Autodesk Fusion 360 part; units mm, degrees
(part 2 of 4)
sketch "Sketch2" plane through (-153, -3, 890) normal (0, -1, 0) x (1, 0, 0)
  circle A0 centre (0, 0) radius 2.75
  circle A1 centre (0, 0) radius 2.75
  circle A2 centre (81, 0) radius 2.75
  circle A3 centre (81, 0) radius 2.75
  circle A4 centre (162, 0) radius 2.75
  circle A5 centre (243, 0) radius 2.75
  circle A6 centre (243, 0) radius 2.75
  circle A7 centre (162, 0) radius 2.75
  circle A8 centre (405, 0) radius 2.75
  circle A9 centre (405, 0) radius 2.75
  circle A10 centre (324, 0) radius 2.75
  circle A11 centre (324, 0) radius 2.75
  circle A12 centre (486, 0) radius 2.75
  circle A13 centre (486, 0) radius 2.75
  circle A14 centre (405, -81) radius 2.75
  circle A15 centre (81, -81) radius 2.75
  circle A16 centre (486, -81) radius 2.75
  circle A17 centre (405, -81) radius 2.75
  circle A18 centre (0, -81) radius 2.75
  circle A19 centre (0, -81) radius 2.75
  circle A20 centre (81, -81) radius 2.75
  circle A21 centre (324, -81) radius 2.75
  circle A22 centre (243, -81) radius 2.75
  circle A23 centre (486, -81) radius 2.75
  circle A24 centre (243, -81) radius 2.75
  circle A25 centre (324, -81) radius 2.75
  circle A26 centre (162, -81) radius 2.75
  circle A27 centre (162, -81) radius 2.75
  circle A28 centre (162, -162) radius 2.75
  circle A29 centre (162, -243) radius 2.75
  circle A30 centre (81, -243) radius 2.75
  circle A31 centre (162, -162) radius 2.75
  circle A32 centre (162, -243) radius 2.75
  circle A33 centre (324, -243) radius 2.75
  circle A34 centre (81, -162) radius 2.75
  circle A35 centre (324, -162) radius 2.75
  circle A36 centre (243, -243) radius 2.75
  circle A37 centre (405, -162) radius 2.75
  circle A38 centre (486, -243) radius 2.75
  circle A39 centre (81, -162) radius 2.75
  circle A40 centre (81, -243) radius 2.75
  circle A41 centre (405, -243) radius 2.75
  circle A42 centre (0, -162) radius 2.75
  circle A43 centre (243, -162) radius 2.75
  circle A44 centre (405, -162) radius 2.75
  circle A45 centre (486, -162) radius 2.75
  circle A46 centre (0, -243) radius 2.75
  circle A47 centre (486, -162) radius 2.75
  circle A48 centre (243, -162) radius 2.75
  circle A49 centre (0, -162) radius 2.75
  circle A50 centre (0, -243) radius 2.75
  circle A51 centre (243, -243) radius 2.75
  circle A52 centre (324, -162) radius 2.75
  circle A53 centre (405, -243) radius 2.75
  circle A54 centre (324, -243) radius 2.75
  circle A55 centre (486, -243) radius 2.75
  circle A56 centre (486, -324) radius 2.75
  circle A57 centre (243, -324) radius 2.75
  circle A58 centre (405, -324) radius 2.75
  circle A59 centre (81, -324) radius 2.75
  circle A60 centre (324, -324) radius 2.75
  circle A61 centre (0, -324) radius 2.75
  circle A62 centre (405, -324) radius 2.75
  circle A63 centre (486, -324) radius 2.75
  circle A64 centre (81, -324) radius 2.75
  circle A65 centre (162, -324) radius 2.75
  circle A66 centre (243, -324) radius 2.75
  circle A67 centre (162, -324) radius 2.75
  circle A68 centre (324, -324) radius 2.75
  circle A69 centre (0, -324) radius 2.75
  point P0 (81, 0)
  point P1 (81, 0)
  point P2 (162, 0)
  point P3 (243, 0)
  point P4 (324, 0)
  point P5 (405, 0)
  point P6 (486, 0)
  point P7 (162, 0)
  point P8 (243, 0)
  point P9 (243, 0)
  point P10 (324, 0)
  point P11 (405, 0)
  point P12 (405, 0)
  point P13 (324, 0)
  point P14 (405, 0)
  point P15 (486, 0)
  point P16 (486, 0)
  point P17 (486, 0)
  point P18 (486, 0)
  point P19 (0, -81)
  point P20 (0, -162)
  point P21 (0, -243)
  point P22 (0, -324)
  point P23 (162, -81)
  point P24 (243, -81)
  point P25 (0, -81)
  point P26 (243, -81)
  point P27 (324, -81)
  point P28 (405, -81)
  point P29 (81, -81)
  point P30 (486, -81)
  point P31 (324, -81)
  point P32 (405, -81)
  point P33 (405, -81)
  point P34 (324, -81)
  point P35 (162, -81)
  point P36 (243, -81)
  point P37 (486, -81)
  point P38 (486, -81)
  point P39 (486, -81)
  point P40 (486, -81)
  point P41 (405, -81)
  point P42 (81, -81)
  point P43 (405, -243)
  point P44 (324, -243)
  point P45 (243, -243)
  point P46 (405, -243)
  point P47 (486, -243)
  point P48 (486, -243)
  point P49 (162, -243)
  point P50 (324, -243)
  point P51 (81, -243)
  point P52 (81, -243)
  point P53 (162, -243)
  point P54 (405, -243)
  point P55 (405, -243)
  point P56 (243, -243)
  point P57 (0, -243)
  point P58 (324, -243)
  point P59 (486, -243)
  point P60 (486, -243)
  point P61 (486, -243)
  point P62 (243, -243)
  point P63 (162, -162)
  point P64 (243, -162)
  point P65 (0, -162)
  point P66 (243, -162)
  point P67 (324, -162)
  point P68 (0, -243)
  point P69 (405, -162)
  point P70 (81, -162)
  point P71 (486, -162)
  point P72 (324, -162)
  point P73 (405, -162)
  point P74 (405, -162)
  point P75 (324, -162)
  point P76 (162, -162)
  point P77 (243, -162)
  point P78 (486, -162)
  point P79 (486, -162)
  point P80 (486, -162)
  point P81 (486, -162)
  point P82 (405, -162)
  point P83 (81, -162)
  point P84 (0, -324)
  point P85 (0, -324)
  point P86 (486, -324)
  point P87 (0, -324)
  point P88 (162, -324)
  point P89 (81, -324)
  point P90 (486, -324)
  point P91 (486, -324)
  point P92 (243, -324)
  point P93 (405, -324)
  point P94 (486, -324)
  point P95 (162, -324)
  point P96 (81, -324)
  point P97 (405, -324)
  point P98 (243, -324)
  point P99 (324, -324)
  point P100 (486, -324)
  point P101 (324, -324)
  point P102 (405, -324)
  point P103 (324, -324)
  point P104 (405, -324)
  point P105 (243, -324)
  dimension "d286" = 5.5
  dimension "d287" = 5.5
  dimension "d288" = 5.5
  dimension "d289" = 5.5
  dimension "d290" = 5.5
  dimension "d291" = 5.5
  dimension "d292" = 5.5
  dimension "d293" = 5.5
  dimension "d294" = 5.5
  dimension "d295" = 5.5
  dimension "d296" = 5.5
  dimension "d297" = 5.5
  dimension "d298" = 5.5
  dimension "d299" = 5.5
  dimension "d300" = 5.5
  dimension "d301" = 5.5
  dimension "d302" = 5.5
  dimension "d303" = 5.5
  dimension "d304" = 5.5
  dimension "d305" = 5.5
  dimension "d306" = 5.5
  dimension "d307" = 5.5
  dimension "d308" = 5.5
  dimension "d309" = 5.5
  dimension "d310" = 5.5
  dimension "d311" = 5.5
  dimension "d312" = 5.5
  dimension "d313" = 5.5
  dimension "d314" = 5.5
  dimension "d315" = 5.5
  dimension "d316" = 5.5
  dimension "d317" = 5.5
  dimension "d318" = 5.5
  dimension "d319" = 5.5
  dimension "d320" = 5.5
  dimension "d321" = 5.5
  dimension "d322" = 5.5
  dimension "d323" = 5.5
  dimension "d324" = 5.5
  dimension "d325" = 5.5
  dimension "d326" = 5.5
  dimension "d327" = 5.5
  dimension "d328" = 5.5
  dimension "d329" = 5.5
  dimension "d330" = 5.5
  dimension "d331" = 5.5
  dimension "d332" = 5.5
  dimension "d333" = 5.5
  dimension "d334" = 5.5
  dimension "d335" = 5.5
  dimension "d336" = 5.5
  dimension "d337" = 5.5
  dimension "d338" = 5.5
  dimension "d339" = 5.5
  dimension "d340" = 5.5
  dimension "d341" = 5.5
  dimension "d342" = 5.5
  dimension "d343" = 5.5
  dimension "d344" = 5.5
  dimension "d345" = 5.5
  dimension "d346" = 5.5
  dimension "d347" = 5.5
  dimension "d348" = 5.5
  dimension "d349" = 5.5
  dimension "d350" = 5.5
  dimension "d351" = 5.5
  dimension "d352" = 5.5
  dimension "d353" = 5.5
  dimension "d354" = 5.5
  dimension "d355" = 5.5
  constraint coincident A0.centre A1.centre
  constraint coincident P1 P0
  constraint coincident P7 P2
  constraint coincident P9 P8
  constraint coincident P13 P10
  constraint coincident P14 P12
  constraint coincident P18 P17
  constraint coincident P25 P19
  constraint coincident P42 P29
  constraint coincident P35 P23
  constraint coincident P36 P26
  constraint coincident P34 P31
  constraint coincident P41 P33
  constraint coincident P40 P39
  constraint coincident P65 P20
  constraint coincident P83 P70
  constraint coincident P76 P63
  constraint coincident P77 P66
  constraint coincident P75 P72
  constraint coincident P82 P74
  constraint coincident P81 P80
  constraint coincident P68 P57
  constraint coincident P52 P51
  constraint coincident P53 P49
  constraint coincident P62 P56
  constraint coincident P58 P50
  constraint coincident P55 P54
  constraint coincident P61 P60
  constraint coincident P87 P85
  constraint coincident P96 P89
  constraint coincident P95 P88
  constraint coincident P105 P98
  constraint coincident P103 P101
  constraint coincident P104 P102
  constraint coincident P100 P94
  measures "d286" diameter of A0
  measures "d287" diameter of A1
  measures "d288" diameter of A2
  measures "d289" diameter of A3
  measures "d290" diameter of A7
  measures "d291" diameter of A4
  measures "d292" diameter of A6
  measures "d293" diameter of A5
  measures "d294" diameter of A10
  measures "d295" diameter of A11
  measures "d296" diameter of A8
  measures "d297" diameter of A9
  measures "d298" diameter of A12
  measures "d299" diameter of A13
  measures "d300" diameter of A19
  measures "d301" diameter of A18
  measures "d302" diameter of A15
  measures "d303" diameter of A20
  measures "d304" diameter of A27
  measures "d305" diameter of A26
  measures "d306" diameter of A24
  measures "d307" diameter of A22
  measures "d308" diameter of A25
  measures "d309" diameter of A21
  measures "d310" diameter of A14
  measures "d311" diameter of A17
  measures "d312" diameter of A16
  measures "d313" diameter of A23
  measures "d314" diameter of A42
  measures "d315" diameter of A49
  measures "d316" diameter of A39
  measures "d317" diameter of A34
  measures "d318" diameter of A28
  measures "d319" diameter of A31
  measures "d320" diameter of A43
  measures "d321" diameter of A48
  measures "d322" diameter of A52
  measures "d323" diameter of A35
  measures "d324" diameter of A37
  measures "d325" diameter of A44
  measures "d326" diameter of A47
  measures "d327" diameter of A45
  measures "d328" diameter of A50
  measures "d329" diameter of A46
  measures "d330" diameter of A40
  measures "d331" diameter of A30
  measures "d332" diameter of A32
  measures "d333" diameter of A29
  measures "d334" diameter of A51
  measures "d335" diameter of A36
  measures "d336" diameter of A33
  measures "d337" diameter of A54
  measures "d338" diameter of A41
  measures "d339" diameter of A53
  measures "d340" diameter of A55
  measures "d341" diameter of A38
  measures "d342" diameter of A69
  measures "d343" diameter of A61
  measures "d344" diameter of A59
  measures "d345" diameter of A64
  measures "d346" diameter of A67
  measures "d347" diameter of A65
  measures "d348" diameter of A57
  measures "d349" diameter of A66
  measures "d350" diameter of A68
  measures "d351" diameter of A60
  measures "d352" diameter of A62
  measures "d353" diameter of A58
  measures "d354" diameter of A56
  measures "d355" diameter of A63
extrude "Extrude2" [suppressed]

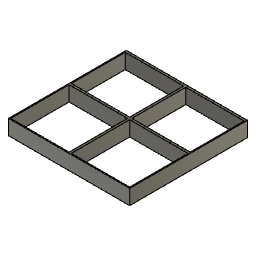
design "Grilla A."
Autodesk Fusion 360 part; units mm, degrees
ref_plane "WorkPlane1" through (0, 0, 0) normal (0, 0, 1) x (1, 0, 0)
sketch "Sketch1" plane through (0, 0, 0) normal (0, 0, 1) x (1, 0, 0)
  line L0 (39, 36.035) -> (-39, 36.035)
  line L1 (-39, 36.035) -> (-39, -36.035)
  line L2 (-39, -36.035) -> (39, -36.035)
  line L3 (39, -36.035) -> (39, 36.035)
  line L4 (39, 36.035) -> (-39, -36.035) construction
  line L5 (-39, 36.035) -> (39, -36.035) construction
  line L6 (-39, -36.035) -> (39, -36.035)
  line L7 (39, -39.035) -> (-39, -39.035)
  line L8 (-39, -39.035) -> (39, -39.035)
  line L9 (39, -39.035) -> (39, -117.035)
  line L10 (39, -117.035) -> (-39, -117.035)
  line L11 (-39, -117.035) -> (-39, -39.035)
  line L12 (120, 36.035) -> (42, -36.035) construction
  line L13 (120, -39.035) -> (120, -117.035)
  line L14 (42, -36.035) -> (120, -36.035)
  line L15 (42, -39.035) -> (120, -39.035)
  line L16 (120, -39.035) -> (42, -39.035)
  line L17 (120, -117.035) -> (42, -117.035)
  line L18 (42, -36.035) -> (120, -36.035)
  line L19 (42, -117.035) -> (42, -39.035)
  line L20 (120, 36.035) -> (42, 36.035)
  line L21 (42, 36.035) -> (42, -36.035)
  line L22 (120, -36.035) -> (120, 36.035)
  line L23 (42, 36.035) -> (120, -36.035) construction
  line L24 (120, 39.035) -> (-39, 39.035)
  line L25 (-39, 39.035) -> (-40.5, 39.035)
  line L26 (-40.5, 39.035) -> (-40.5, -117.035)
  line L27 (120, 39.035) -> (121.5, 39.035)
  line L28 (121.5, 39.035) -> (121.5, -117.035)
  line L29 (121.5, -117.035) -> (121.5, -118.535)
  line L30 (121.5, -118.535) -> (-40.5, -118.535)
  line L31 (-40.5, -118.535) -> (-40.5, -117.035)
  line L32 (-39, 36.035) -> (39, 36.035)
  line L33 (42, 36.035) -> (120, 36.035)
  line L34 (-39, -117.035) -> (-39, -39.035)
  line L35 (-39, -36.035) -> (-39, 36.035)
  line L36 (39, -117.035) -> (39, -39.035)
  line L37 (39, -36.035) -> (39, 36.035)
  line L38 (42, 36.035) -> (42, -36.035)
  line L39 (42, -39.035) -> (42, -117.035)
  line L40 (120, -117.035) -> (120, -39.035)
  line L41 (120, -36.035) -> (120, 36.035)
  line L42 (-39, -117.035) -> (39, -117.035)
  line L43 (42, -117.035) -> (120, -117.035)
  point P0 (81, 0)
  point P1 (81, 0)
  dimension "d55" = 78
  dimension "d56" = 72.07
  dimension "d57" = 3
  dimension "d58" = 78
  dimension "d59" = 78
  dimension "d60" = 78
  dimension "d61" = 72.07
  dimension "d62" = 3
  dimension "d63" = 78
  dimension "d64" = 78
  dimension "d65" = 3
  dimension "d66" = 3
  dimension "d67" = 1.5
  dimension "d68" = 1.5
  dimension "d69" = 1.5
  constraint horizontal L0
  constraint perpendicular L0 L1
  constraint parallel L0 L2
  constraint parallel L1 L3
  constraint coincident L4 origin
  constraint coincident L5 origin
  constraint horizontal L6
  constraint horizontal L7
  constraint horizontal L8
  constraint vertical L9
  constraint horizontal L10
  constraint vertical L11
  constraint horizontal L20
  constraint perpendicular L20 L21
  constraint parallel L18 L20
  constraint parallel L21 L22
  constraint coincident P1 L12
  constraint coincident P1 L23
  constraint coincident P1 P0
  constraint horizontal L14
  constraint horizontal L16
  constraint horizontal L15
  constraint vertical L13
  constraint horizontal L17
  constraint vertical L19
  constraint vertical L38
  constraint vertical L36
  constraint horizontal L32
  constraint horizontal L24
  constraint horizontal L25
  constraint vertical L26
  constraint vertical L34
  constraint horizontal L27
  constraint vertical L28
  constraint vertical L40
  constraint horizontal L42
  constraint vertical L29
  constraint horizontal L30
  constraint vertical L31
  constraint collinear L32 L33
  constraint collinear L34 L35
  constraint collinear L36 L37
  constraint collinear L38 L39
  constraint collinear L40 L41
  constraint collinear L42 L43
  measures "d55" distance of L1.end L2.end
  measures "d56" distance of L0.end L1.end
  measures "d57" distance of L1.end L7.end
  measures "d58" distance of L7.end L7.start
  measures "d59" distance of L7.end L10.end
  measures "d60" distance of L12.end L14.end
  measures "d61" distance of L20.end L12.end
  measures "d62" distance of L12.end L15.start
  measures "d63" distance of L15.start L13.start
  measures "d64" distance of L15.start L17.end
  measures "d65" distance of L0.start L20.end
  measures "d66" distance of L0.end L24.end
  measures "d67" distance of L24.end L25.end
  measures "d68" distance of L24.start L27.end
  measures "d69" distance of L26.end L30.end
extrude "Extrude2" add sketch "Sketch1" along normal blind 20

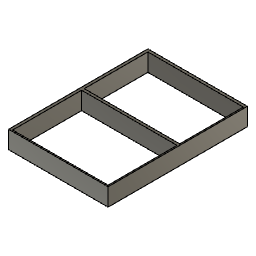
design "C Grilla"
Autodesk Fusion 360 part; units mm, degrees
sketch "Sketch1" plane through (0, 0, 0) normal (0, 0, 1) x (1, 0, 0)
  line L0 (54, 36) -> (-54, 36)
  line L1 (-54, 36) -> (-54, -36)
  line L2 (-54, -36) -> (54, -36)
  line L3 (54, -36) -> (54, 36)
  line L4 (54, 36) -> (-54, -36) construction
  line L5 (-54, 36) -> (54, -36) construction
  line L6 (-54, -39) -> (54, -39)
  line L7 (55.5, 39) -> (-57, 39)
  line L8 (-57, 39) -> (-57, -39)
  line L9 (-54, -39) -> (54, -39)
  line L10 (54, -39) -> (54, -117)
  line L11 (54, -117) -> (-54, -117)
  line L12 (-54, -117) -> (-54, -39)
  line L13 (-57, -39) -> (-57, -118.5)
  line L14 (55.5, -36) -> (55.5, 36)
  line L15 (55.5, -39) -> (55.5, -118.5)
  line L16 (55.5, -118.5) -> (-54, -118.5)
  line L17 (55.5, -36) -> (55.5, -39)
  line L18 (55.5, 36) -> (55.5, 39)
  line L19 (-54, -118.5) -> (-57, -118.5)
  dimension "d13" = 108
  dimension "d14" = 72
  dimension "d16" = 108
  dimension "d17" = 78
  dimension "d18" = 1.5
  dimension "d19" = -1.5
  constraint horizontal L0
  constraint perpendicular L0 L1
  constraint parallel L0 L2
  constraint parallel L1 L3
  constraint coincident L4 origin
  constraint coincident L5 origin
  constraint horizontal L9
  constraint vertical L10
  constraint horizontal L11
  constraint vertical L12
  constraint coincident L6.start L9.start
  constraint perpendicular L11 L13
  constraint parallel L2 L6
  constraint parallel L0 L7
  constraint parallel L1 L8
  constraint parallel L15 L17
  constraint perpendicular L7 L18
  constraint perpendicular L13 L19
  measures "d13" distance of L1.end L2.end
  measures "d14" distance of L0.end L1.end
  measures "d16" distance of L6.start L6.end
  measures "d17" distance of L6.start L11.end
extrude "Extrude2" add sketch "Sketch1" along normal blind 20

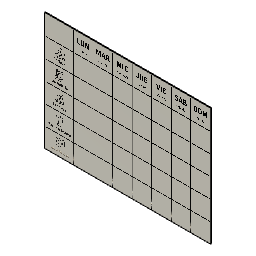
design "pantalla render"
Autodesk Fusion 360 part; units mm, degrees
sketch "Sketch1" plane through (0, 0, 0) normal (0, 1, 0) x (1, 0, 0)
  line L0 (340.5, 241.5) -> (-340.5, 241.5)
  line L1 (-340.5, 241.5) -> (-340.5, -241.5)
  line L2 (-340.5, -241.5) -> (340.5, -241.5)
  line L3 (340.5, -241.5) -> (340.5, 241.5)
  line L4 (340.5, 241.5) -> (-340.5, -241.5) construction
  line L5 (-340.5, 241.5) -> (340.5, -241.5) construction
  dimension "d1" = 681
  dimension "d2" = 483
  constraint horizontal L0
  constraint perpendicular L0 L1
  constraint parallel L0 L2
  constraint parallel L1 L3
  constraint coincident L4 origin
  constraint coincident L5 origin
  measures "d1" distance of L1.end L2.end
  measures "d2" distance of L0.end L1.end
extrude "Extrude1" add sketch "Sketch1" against normal blind 3

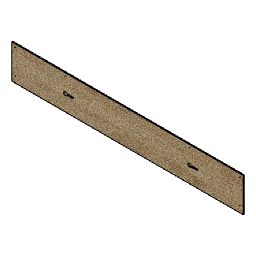
design "Pieza trasera fondo"
Autodesk Fusion 360 part; units mm, degrees
sketch "Sketch1" plane through (0, 0, 0) normal (0, 1, 0) x (1, 0, 0)
  arc A0 (187.942, -190.4984) -> (187.4765, -190.7709) centre (187.922, -190.998) ccw
  line L0 (340.5, -50) -> (337.5, -50)
  line L1 (-161.02, -186.5) -> (-178.0217, -186.5)
  circle A1 centre (330.5, -232.5) radius 1
  line L2 (188.022, -190.5) -> (205.0238, -190.5)
  line L3 (-337.5, -238.5) -> (-340.5, -238.5)
  circle A2 centre (183.022, -233.5) radius 1
  arc A3 (187.942, -190.4984) -> (188.022, -190.5) centre (188.022, -188.5) ccw
  line L4 (50, -238.5) -> (50, -241.5)
  line L5 (-337.5, -238.5) -> (-337.5, -241.5)
  arc A4 (187.4765, -186.2291) -> (187.942, -186.5016) centre (187.922, -186.002) ccw
  circle A5 centre (-183.0217, -233.5) radius 1
  circle A6 centre (328.5, 226.5) radius 1
  circle A7 centre (330.5, -159.5) radius 1
  circle A8 centre (-330.5, -232.5) radius 1
  line L6 (50, 238.5) -> (337.5, 238.5)
  line L7 (-337.5, 50) -> (-337.5, 238.5)
  circle A9 centre (-330.5, -159.3463) radius 1
  line L8 (-50, -241.5) -> (-50, -238.5)
  circle A10 centre (-328.5, 226.5) radius 1
  line L9 (-340.5, -241.5) -> (340.5, -241.5)
  line L10 (-178.0217, -186.5) -> (-178.5672, -186.2291)
  line L11 (337.5, -238.5) -> (50, -238.5)
  line L12 (340.5, 50) -> (340.5, -50)
  line L13 (-337.5, -50) -> (-340.5, -50)
  line L14 (-50, -238.5) -> (-337.5, -238.5)
  line L15 (29.8496, 241.5) -> (50, 241.5)
  arc A11 (-161.02, -190.5) -> (-161.02, -186.5) centre (-161.02, -188.5) ccw
  line L16 (-340.5, -141.5) -> (-340.5, -241.5)
  line L17 (337.5, 50) -> (340.5, 50)
  line L18 (-340.5, 50) -> (-337.5, 50)
  circle A12 centre (183.0674, 231.5957) radius 1
  line L19 (340.5, -241.5) -> (340.5, -141.5)
  line L20 (-50, 241.5) -> (-29.8496, 241.5)
  line L21 (337.5, 238.5) -> (337.5, 50)
  line L22 (-50, 238.5) -> (-50, 241.5)
  circle A13 centre (-182.9674, 230.6288) radius 1
  line L23 (337.5, -238.5) -> (340.5, -238.5)
  circle A14 centre (326.5, -2.556) radius 1
  line L24 (50, -241.5) -> (-50, -241.5)
  line L25 (-337.5, -238.5) -> (-337.5, -50)
  arc A15 (187.4765, -186.2291) -> (187.4765, -190.7709) centre (183.022, -188.5) ccw
  line L26 (205.0238, -186.5) -> (188.022, -186.5)
  line L27 (340.5, -141.5) -> (-340.5, -141.5)
  line L28 (-178.5672, -190.7709) -> (-178.0217, -190.5)
  line L29 (-340.5, -50) -> (-340.5, 50)
  line L30 (-178.0217, -190.5) -> (-161.02, -190.5)
  line L31 (337.5, -50) -> (337.5, -238.5)
  arc A16 (205.0238, -190.5) -> (205.0238, -186.5) centre (205.0238, -188.5) ccw
  line L32 (-337.5, 238.5) -> (-50, 238.5)
  arc A17 (-29.8496, 241.5) -> (29.8496, 241.5) centre (0, 238.5) ccw
  arc A18 (188.022, -186.5) -> (187.942, -186.5016) centre (188.022, -188.5) ccw
  arc A19 (-178.5672, -186.2291) -> (-178.5672, -190.7709) centre (-183.0217, -188.5) ccw
  line L33 (50, 241.5) -> (50, 238.5)
  dimension "d32" = 82.1537
  dimension "d33" = 157.4783
  measures "d32" distance of A9.centre L9
  measures "d33" distance of A5.centre L16
extrude "Extrude1" add sketch "Sketch1" along normal blind 3 contours L4 L8 L9 L11 L14 L24 L25 L27 L31 | L19 L23 L27 L31 | L3 L16 L25 L27 | L4 L9 L11 L19 L23 | L3 L5 L9 L16 | L5 L8 L9 L14

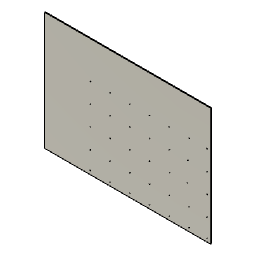
design "A. Pantalla delantera"
Autodesk Fusion 360 part; units mm, degrees
ref_plane "WorkPlane1" through (0, 0, 0) normal (0, 1, 0) x (0, 0, 1)
sketch "Sketch2" plane through (0, 0, 0) normal (0, 1, 0) x (1, 0, 0)
  line L0 (340.5, -241.5) -> (-340.5, -241.5)
  line L1 (-340.5, -241.5) -> (-340.5, 241.5)
  line L2 (-340.5, 241.5) -> (340.5, 241.5)
  line L3 (340.5, 241.5) -> (340.5, -241.5)
  line L4 (340.5, -241.5) -> (-340.5, 241.5) construction
  line L5 (-340.5, -241.5) -> (340.5, 241.5) construction
  dimension "d6" = 681
  dimension "d7" = 483
  constraint horizontal L0
  constraint perpendicular L0 L1
  constraint parallel L0 L2
  constraint parallel L1 L3
  constraint coincident L4 origin
  constraint coincident L5 origin
  measures "d6" distance of L1.end L2.end
  measures "d7" distance of L0.end L1.end
extrude "Extrude2" add sketch "Sketch2" along normal blind 3
ref_plane "WorkPlane2" through (0, 0, 0) normal (0, -1, 0) x (-1, 0, 0)
sketch "Sketch3" plane through (0, 0, 0) normal (0, -1, 0) x (1, 0, 0)
  line L0 (-340.5, -241.5) -> (340.5, -241.5) construction
  line L1 (340.5, -241.5) -> (340.5, 241.5) construction
  line L2 (340.5, 241.5) -> (-340.5, 241.5) construction
  line L3 (-340.5, 241.5) -> (-340.5, -241.5) construction
  line L4 (-340.5, 241.5) -> (-226.5, 241.5) construction
  line L5 (-226.5, 241.5) -> (-226.5, -241.5) construction
  line L6 (-226.5, -241.5) -> (-340.5, -241.5) construction
  line L7 (-340.5, -241.5) -> (-340.5, 241.5) construction
  line L8 (-226.5, 241.5) -> (-223.5, 241.5) construction
  line L9 (-223.5, 241.5) -> (-223.5, -241.5) construction
  line L10 (-223.5, -241.5) -> (-226.5, -241.5)
  line L11 (-226.5, -241.5) -> (-226.5, 241.5) construction
  line L12 (-223.5, 241.5) -> (-145.5, 241.5) construction
  line L13 (-145.5, 241.5) -> (-145.5, 163.5) construction
  line L14 (-145.5, 163.5) -> (-223.5, 163.5)
  line L15 (-223.5, 163.5) -> (-223.5, 241.5) construction
  line L16 (-145.5, 241.5) -> (-142.5, 241.5) construction
  line L17 (-142.5, 241.5) -> (-142.5, -234) construction
  line L18 (-142.5, -234) -> (-145.5, -234)
  line L19 (-145.5, -234) -> (-145.5, 241.5) construction
  line L20 (-142.5, 241.5) -> (-64.5, 241.5) construction
  line L21 (-64.5, 241.5) -> (-64.5, 163.5) construction
  line L22 (-64.5, 163.5) -> (-142.5, 163.5)
  line L23 (-142.5, 163.5) -> (-142.5, 241.5) construction
  line L24 (-64.5, 241.5) -> (-61.5, 241.5) construction
  line L25 (-61.5, 241.5) -> (-61.5, -241.5) construction
  line L26 (-61.5, -241.5) -> (-64.5, -241.5)
  line L27 (-64.5, -241.5) -> (-64.5, 241.5) construction
  line L28 (-61.5, 241.5) -> (16.5, 241.5) construction
  line L29 (16.5, 241.5) -> (16.5, 163.5) construction
  line L30 (16.5, 163.5) -> (-61.5, 163.5)
  line L31 (-61.5, 163.5) -> (-61.5, 241.5) construction
  line L32 (16.5, 241.5) -> (19.5, 241.5) construction
  line L33 (19.5, 241.5) -> (19.5, -241.5) construction
  line L34 (19.5, -241.5) -> (16.5, -241.5)
  line L35 (16.5, -241.5) -> (16.5, 241.5) construction
  line L36 (19.5, 241.5) -> (97.5, 241.5) construction
  line L37 (97.5, 241.5) -> (97.5, 163.5) construction
  line L38 (97.5, 163.5) -> (19.5, 163.5)
  line L39 (19.5, 163.5) -> (19.5, 241.5) construction
  line L40 (97.5, 241.5) -> (100.5, 241.5) construction
  line L41 (100.5, 241.5) -> (100.5, -241.5) construction
  line L42 (100.5, -241.5) -> (97.5, -241.5)
  line L43 (97.5, -241.5) -> (97.5, 241.5) construction
  line L44 (100.5, 241.5) -> (178.5, 241.5) construction
  line L45 (178.5, 241.5) -> (178.5, 163.5) construction
  line L46 (178.5, 163.5) -> (100.5, 163.5)
  line L47 (100.5, 163.5) -> (100.5, 241.5) construction
  line L48 (178.5, 241.5) -> (181.5, 241.5) construction
  line L49 (181.5, 241.5) -> (181.5, -241.5) construction
  line L50 (181.5, -241.5) -> (178.5, -241.5)
  line L51 (178.5, -241.5) -> (178.5, 241.5) construction
  line L52 (181.5, 241.5) -> (259.5, 241.5) construction
  line L53 (259.5, 241.5) -> (259.5, 163.5) construction
  line L54 (259.5, 163.5) -> (181.5, 163.5)
  line L55 (181.5, 163.5) -> (181.5, 241.5) construction
  line L56 (259.5, 241.5) -> (262.5, 241.5) construction
  line L57 (262.5, 241.5) -> (262.5, -241.5) construction
  line L58 (262.5, -241.5) -> (259.5, -241.5)
  line L59 (259.5, -241.5) -> (259.5, 241.5) construction
  line L60 (262.5, 241.5) -> (340.5, 241.5) construction
  line L61 (340.5, 241.5) -> (340.5, 163.5) construction
  line L62 (340.5, 163.5) -> (262.5, 163.5)
  line L63 (262.5, 163.5) -> (262.5, 241.5) construction
  line L64 (340.5, 163.5) -> (-340.5, 163.5) construction
  line L65 (-340.5, 163.5) -> (-340.5, 160.5)
  line L66 (-340.5, 160.5) -> (340.5, 160.5) construction
  line L67 (340.5, 160.5) -> (340.5, 163.5)
  line L68 (340.5, 160.5) -> (-340.5, 160.5) construction
  line L69 (-340.5, 160.5) -> (-340.5, 82.5)
  line L70 (-340.5, 82.5) -> (340.5, 82.5) construction
  line L71 (340.5, 82.5) -> (340.5, 160.5)
  line L72 (340.5, 82.5) -> (-340.5, 82.5) construction
  line L73 (-340.5, 82.5) -> (-340.5, 79.5)
  line L74 (-340.5, 79.5) -> (340.5, 79.5) construction
  line L75 (340.5, 79.5) -> (340.5, 82.5)
  line L76 (340.5, 79.5) -> (-340.5, 79.5) construction
  line L77 (-340.5, 79.5) -> (-340.5, 1.5)
  line L78 (-340.5, 1.5) -> (340.5, 1.5) construction
  line L79 (340.5, 1.5) -> (340.5, 79.5)
  line L80 (340.5, 1.5) -> (-340.5, 1.5) construction
  line L81 (-340.5, 1.5) -> (-340.5, -1.5)
  line L82 (-340.5, -1.5) -> (340.5, -1.5) construction
  line L83 (340.5, -1.5) -> (340.5, 1.5)
  line L84 (340.5, -1.5) -> (-340.5, -1.5) construction
  line L85 (-340.5, -1.5) -> (-340.5, -79.5)
  line L86 (-340.5, -79.5) -> (340.5, -79.5) construction
  line L87 (340.5, -79.5) -> (340.5, -1.5)
  line L88 (340.5, -79.5) -> (-340.5, -79.5) construction
  line L89 (-340.5, -79.5) -> (-340.5, -82.5)
  line L90 (-340.5, -82.5) -> (340.5, -82.5) construction
  line L91 (340.5, -82.5) -> (340.5, -79.5)
  line L92 (340.5, -82.5) -> (-340.5, -82.5) construction
  line L93 (-340.5, -82.5) -> (-340.5, -160.5)
  line L94 (-340.5, -160.5) -> (340.5, -160.5) construction
  line L95 (340.5, -160.5) -> (340.5, -82.5)
  line L96 (340.5, -160.5) -> (-340.5, -160.5) construction
  line L97 (-340.5, -160.5) -> (-340.5, -163.5)
  line L98 (-340.5, -163.5) -> (340.5, -163.5) construction
  line L99 (340.5, -163.5) -> (340.5, -160.5)
  line L100 (-145.5, 82.5) -> (-160.5, 82.5)
  line L101 (-160.5, 82.5) -> (-160.5, 97.5)
  line L102 (-160.5, 97.5) -> (-145.5, 97.5)
  line L103 (-145.5, 97.5) -> (-145.5, 82.5)
  line L104 (-64.5, 82.5) -> (-79.5, 82.5)
  line L105 (-79.5, 82.5) -> (-79.5, 97.5)
  line L106 (-79.5, 97.5) -> (-64.5, 97.5)
  line L107 (-64.5, 97.5) -> (-64.5, 82.5)
  line L108 (16.5, 82.5) -> (1.5, 82.5)
  line L109 (1.5, 82.5) -> (1.5, 97.5)
  line L110 (1.5, 97.5) -> (16.5, 97.5)
  line L111 (16.5, 97.5) -> (16.5, 82.5)
  line L112 (-145.5, 1.5) -> (-160.5, 1.5)
  line L113 (-160.5, 1.5) -> (-160.5, 16.5)
  line L114 (-160.5, 16.5) -> (-145.5, 16.5)
  line L115 (-145.5, 16.5) -> (-145.5, 1.5)
  line L116 (-64.5, 1.5) -> (-79.5, 1.5)
  line L117 (-79.5, 1.5) -> (-79.5, 16.5)
  line L118 (-79.5, 16.5) -> (-64.5, 16.5)
  line L119 (-64.5, 16.5) -> (-64.5, 1.5)
  line L120 (16.5, 1.5) -> (1.5, 1.5)
  line L121 (1.5, 1.5) -> (1.5, 16.5)
  line L122 (1.5, 16.5) -> (16.5, 16.5)
  line L123 (16.5, 16.5) -> (16.5, 1.5)
  line L124 (-145.5, -79.5) -> (-160.5, -79.5)
  line L125 (-160.5, -79.5) -> (-160.5, -64.5)
  line L126 (-160.5, -64.5) -> (-145.5, -64.5)
  line L127 (-145.5, -64.5) -> (-145.5, -79.5)
  line L128 (-145.5, -160.5) -> (-160.5, -160.5)
  line L129 (-160.5, -160.5) -> (-160.5, -145.5)
  line L130 (-160.5, -145.5) -> (-145.5, -145.5)
  line L131 (-145.5, -145.5) -> (-145.5, -160.5)
  line L132 (-64.5, -79.5) -> (-79.5, -79.5)
  line L133 (-79.5, -79.5) -> (-79.5, -64.5)
  line L134 (-79.5, -64.5) -> (-64.5, -64.5)
  line L135 (-64.5, -64.5) -> (-64.5, -79.5)
  line L136 (-64.5, -160.5) -> (-79.5, -160.5)
  line L137 (-79.5, -160.5) -> (-79.5, -145.5)
  line L138 (-79.5, -145.5) -> (-64.5, -145.5)
  line L139 (-64.5, -145.5) -> (-64.5, -160.5)
  line L140 (16.5, -160.5) -> (1.5, -160.5)
  line L141 (1.5, -160.5) -> (1.5, -145.5)
  line L142 (1.5, -145.5) -> (16.5, -145.5)
  line L143 (16.5, -145.5) -> (16.5, -160.5)
  line L144 (16.5, -79.5) -> (1.5, -79.5)
  line L145 (1.5, -79.5) -> (1.5, -64.5)
  line L146 (1.5, -64.5) -> (16.5, -64.5)
  line L147 (16.5, -64.5) -> (16.5, -79.5)
  line L148 (-145.5, -234) -> (-160.5, -234)
  line L149 (-160.5, -234) -> (-160.5, -219)
  line L150 (-160.5, -219) -> (-145.5, -219)
  line L151 (-145.5, -219) -> (-145.5, -234)
  line L152 (-64.5, -241.5) -> (-79.5, -241.5)
  line L153 (-79.5, -241.5) -> (-79.5, -226.5)
  line L154 (-79.5, -226.5) -> (-64.5, -226.5)
  line L155 (-64.5, -226.5) -> (-64.5, -241.5)
  line L156 (16.5, -241.5) -> (1.5, -241.5)
  line L157 (1.5, -241.5) -> (1.5, -226.5)
  line L158 (1.5, -226.5) -> (16.5, -226.5)
  line L159 (16.5, -226.5) -> (16.5, -241.5)
  line L160 (97.5, 82.5) -> (82.5, 82.5)
  line L161 (82.5, 82.5) -> (82.5, 97.5)
  line L162 (82.5, 97.5) -> (97.5, 97.5)
  line L163 (97.5, 97.5) -> (97.5, 82.5)
  line L164 (178.5, 82.5) -> (163.5, 82.5)
  line L165 (163.5, 82.5) -> (163.5, 97.5)
  line L166 (163.5, 97.5) -> (178.5, 97.5)
  line L167 (178.5, 97.5) -> (178.5, 82.5)
  line L168 (259.5, 82.5) -> (244.5, 82.5)
  line L169 (244.5, 82.5) -> (244.5, 97.5)
  line L170 (244.5, 97.5) -> (259.5, 97.5)
  line L171 (259.5, 97.5) -> (259.5, 82.5)
  line L172 (97.5, 1.5) -> (82.5, 1.5)
  line L173 (82.5, 1.5) -> (82.5, 16.5)
  line L174 (82.5, 16.5) -> (97.5, 16.5)
  line L175 (97.5, 16.5) -> (97.5, 1.5)
  line L176 (178.5, 1.5) -> (163.5, 1.5)
  line L177 (163.5, 1.5) -> (163.5, 16.5)
  line L178 (163.5, 16.5) -> (178.5, 16.5)
  line L179 (178.5, 16.5) -> (178.5, 1.5)
  line L180 (97.5, -79.5) -> (82.5, -79.5)
  line L181 (82.5, -79.5) -> (82.5, -64.5)
  line L182 (82.5, -64.5) -> (97.5, -64.5)
  line L183 (97.5, -64.5) -> (97.5, -79.5)
  line L184 (178.5, -79.5) -> (163.5, -79.5)
  line L185 (163.5, -79.5) -> (163.5, -64.5)
  line L186 (163.5, -64.5) -> (178.5, -64.5)
  line L187 (178.5, -64.5) -> (178.5, -79.5)
  line L188 (97.5, -160.5) -> (82.5, -160.5)
  line L189 (82.5, -160.5) -> (82.5, -145.5)
  line L190 (82.5, -145.5) -> (97.5, -145.5)
  line L191 (97.5, -145.5) -> (97.5, -160.5)
  line L192 (178.5, -160.5) -> (163.5, -160.5)
  line L193 (163.5, -160.5) -> (163.5, -145.5)
  line L194 (163.5, -145.5) -> (178.5, -145.5)
  line L195 (178.5, -145.5) -> (178.5, -160.5)
  line L196 (259.5, -160.5) -> (244.5, -160.5)
  line L197 (244.5, -160.5) -> (244.5, -145.5)
  line L198 (244.5, -145.5) -> (259.5, -145.5)
  line L199 (259.5, -145.5) -> (259.5, -160.5)
  line L200 (259.5, -79.5) -> (244.5, -79.5)
  line L201 (244.5, -79.5) -> (244.5, -64.5)
  line L202 (244.5, -64.5) -> (259.5, -64.5)
  line L203 (259.5, -64.5) -> (259.5, -79.5)
  line L204 (340.5, -79.5) -> (325.5, -79.5)
  line L205 (325.5, -79.5) -> (325.5, -64.5)
  line L206 (325.5, -64.5) -> (340.5, -64.5)
  line L207 (340.5, -64.5) -> (340.5, -79.5)
  line L208 (340.5, -160.5) -> (325.5, -160.5)
  line L209 (325.5, -160.5) -> (325.5, -145.5)
  line L210 (325.5, -145.5) -> (340.5, -145.5)
  line L211 (340.5, -145.5) -> (340.5, -160.5)
  line L212 (259.5, 1.5) -> (244.5, 1.5)
  line L213 (244.5, 1.5) -> (244.5, 16.5)
  line L214 (244.5, 16.5) -> (259.5, 16.5)
  line L215 (259.5, 16.5) -> (259.5, 1.5)
  line L216 (340.5, 1.5) -> (325.5, 1.5)
  line L217 (325.5, 1.5) -> (325.5, 16.5)
  line L218 (325.5, 16.5) -> (340.5, 16.5)
  line L219 (340.5, 16.5) -> (340.5, 1.5)
  line L220 (340.5, 82.5) -> (325.5, 82.5)
  line L221 (325.5, 82.5) -> (325.5, 97.5)
  line L222 (325.5, 97.5) -> (340.5, 97.5)
  line L223 (340.5, 97.5) -> (340.5, 82.5)
  line L224 (97.5, -241.5) -> (82.5, -241.5)
  line L225 (82.5, -241.5) -> (82.5, -226.5)
  line L226 (82.5, -226.5) -> (97.5, -226.5)
  line L227 (97.5, -226.5) -> (97.5, -241.5)
  line L228 (178.5, -241.5) -> (163.5, -241.5)
  line L229 (163.5, -241.5) -> (163.5, -226.5)
  line L230 (163.5, -226.5) -> (178.5, -226.5)
  line L231 (178.5, -226.5) -> (178.5, -241.5)
  line L232 (259.5, -241.5) -> (244.5, -241.5)
  line L233 (244.5, -241.5) -> (244.5, -226.5)
  line L234 (244.5, -226.5) -> (259.5, -226.5)
  line L235 (259.5, -226.5) -> (259.5, -241.5)
  line L236 (340.5, -241.5) -> (325.5, -241.5)
  line L237 (325.5, -241.5) -> (325.5, -226.5)
  line L238 (325.5, -226.5) -> (340.5, -226.5)
  line L239 (340.5, -226.5) -> (340.5, -241.5)
  circle A0 centre (-153, -226.5) radius 1.5
  circle A1 centre (-72, -226.5) radius 1.5
  circle A2 centre (9, -226.5) radius 1.5
  circle A3 centre (90, -226.5) radius 1.5
  circle A4 centre (171, -226.5) radius 1.5
  circle A5 centre (252, -226.5) radius 1.5
  circle A6 centre (325.5, -226.503) radius 1.5
  circle A7 centre (325.5, -153) radius 1.5
  circle A8 centre (252, -153) radius 1.5
  circle A9 centre (171, -153) radius 1.5
  circle A10 centre (90, -153) radius 1.5
  circle A11 centre (9, -153) radius 1.5
  circle A12 centre (-72, -153) radius 1.5
  circle A13 centre (-153, -153) radius 1.5
  circle A14 centre (325.5, -72) radius 1.5
  circle A15 centre (244.5, -72.0337) radius 1.5
  circle A16 centre (171, -72) radius 1.5
  circle A17 centre (90, -72) radius 1.5
  circle A18 centre (9, -72) radius 1.5
  circle A19 centre (-72, -72) radius 1.5
  circle A20 centre (-153, -72) radius 1.5
  circle A21 centre (-153, 90) radius 1.5
  circle A22 centre (-72, 90) radius 1.5
  circle A23 centre (-152.9999, 9) radius 1.5
  circle A24 centre (-72, 9) radius 1.5
  circle A25 centre (9, 90) radius 1.5
  circle A26 centre (9, 9) radius 1.5
  circle A27 centre (90, 90) radius 1.5
  circle A28 centre (90, 9) radius 1.5
  circle A29 centre (171, 90) radius 1.5
  circle A30 centre (171, 9) radius 1.5
  circle A31 centre (252, 90) radius 1.5
  circle A32 centre (246.93, 9) radius 1.5
  circle A33 centre (325.5, 9) radius 1.5
  line L240 (-153, -234) -> (-153, -219)
  line L241 (330.7009, -241.5) -> (330.7009, -226.5)
  line L242 (-153, -226.5) -> (-153, 145)
  line L243 (-145.5, 9) -> (-160.5, 9)
  line L244 (-160.5, -72) -> (-145.5, -72)
  line L245 (-160.5, -153) -> (-145.5, -153)
  line L246 (-153, -226.5) -> (347.6008, -226.5)
  line L247 (325.5, -226.5) -> (325.5, 272.3057)
  circle A34 centre (325.5, 90) radius 1.5
  point P0 (-72, -226.5)
  point P1 (-153, 9)
  point P2 (-153, -72)
  point P3 (-153, -153)
  dimension "d11" = 114
  dimension "d12" = 3
  dimension "d13" = 78
  dimension "d14" = 78
  dimension "d15" = 3
  dimension "d16" = 78
  dimension "d17" = 78
  dimension "d18" = 3
  dimension "d19" = 78
  dimension "d20" = 78
  dimension "d21" = 3
  dimension "d22" = 78
  dimension "d23" = 78
  dimension "d24" = 3
  dimension "d25" = 78
  dimension "d26" = 78
  dimension "d27" = 3
  dimension "d28" = 78
  dimension "d29" = 78
  dimension "d30" = 3
  dimension "d31" = 483
  dimension "d32" = 78
  dimension "d33" = 3
  dimension "d34" = 78
  dimension "d35" = 3
  dimension "d36" = 78
  dimension "d37" = 3
  dimension "d38" = 78
  dimension "d39" = 3
  dimension "d40" = 78
  dimension "d41" = 3
  dimension "d42" = 15
  dimension "d43" = 15
  dimension "d44" = 15
  dimension "d45" = 15
  dimension "d46" = 15
  dimension "d47" = 15
  dimension "d48" = 15
  dimension "d49" = 15
  dimension "d50" = 15
  dimension "d51" = 15
  dimension "d52" = 15
  dimension "d53" = 15
  dimension "d54" = 15
  dimension "d55" = 15
  dimension "d56" = 15
  dimension "d57" = 15
  dimension "d58" = 15
  dimension "d59" = 15
  dimension "d60" = 15
  dimension "d61" = 15
  dimension "d62" = 15
  dimension "d63" = 15
  dimension "d64" = 15
  dimension "d65" = 15
  dimension "d66" = 15
  dimension "d67" = 15
  dimension "d68" = 15
  dimension "d69" = 15
  dimension "d70" = 15
  dimension "d71" = 15
  dimension "d72" = 15
  dimension "d73" = 15
  dimension "d74" = 15
  dimension "d75" = 15
  dimension "d76" = 15
  dimension "d77" = 15
  dimension "d78" = 15
  dimension "d79" = 15
  dimension "d80" = 15
  dimension "d81" = 15
  dimension "d82" = 15
  dimension "d83" = 15
  dimension "d84" = 15
  dimension "d85" = 15
  dimension "d86" = 15
  dimension "d87" = 15
  dimension "d88" = 15
  dimension "d89" = 15
  dimension "d90" = 15
  dimension "d91" = 15
  dimension "d92" = 15
  dimension "d93" = 15
  dimension "d94" = 15
  dimension "d95" = 15
  dimension "d96" = 15
  dimension "d97" = 15
  dimension "d98" = 15
  dimension "d99" = 15
  dimension "d100" = 15
  dimension "d101" = 15
  dimension "d102" = 15
  dimension "d103" = 15
  dimension "d104" = 15
  dimension "d105" = 15
  dimension "d106" = 15
  dimension "d107" = 15
  dimension "d108" = 15
  dimension "d109" = 15
  dimension "d110" = 15
  dimension "d111" = 15
  dimension "d112" = 3
  dimension "d113" = 3
  dimension "d114" = 3
  dimension "d115" = 3
  dimension "d116" = 3
  dimension "d117" = 3
  dimension "d118" = 3
  dimension "d119" = 3
  dimension "d120" = 3
  dimension "d121" = 3
  dimension "d122" = 3
  dimension "d123" = 3
  dimension "d124" = 3
  dimension "d125" = 3
  dimension "d126" = 3
  dimension "d127" = 3
  dimension "d128" = 3
  dimension "d129" = 3
  dimension "d130" = 3
  dimension "d131" = 3
  dimension "d132" = 3
  dimension "d133" = 3
  dimension "d134" = 3
  dimension "d135" = 3
  dimension "d136" = 3
  dimension "d137" = 3
  dimension "d138" = 3
  dimension "d139" = 3
  dimension "d140" = 3
  dimension "d141" = 3
  dimension "d142" = 3
  dimension "d143" = 3
  dimension "d144" = 3
  dimension "d146" = 3
  dimension "d149" = 151.5
  dimension "d150" = 81
  dimension "d151" = 81
  dimension "d152" = 81
  dimension "d154" = 7.5
  dimension "d155" = 187.5
  dimension "d156" = 81
  dimension "d157" = 81
  dimension "d158" = 81
  dimension "d159" = 81
  dimension "d160" = 81
  dimension "d164" = 78.57
  dimension "d167" = 81
  dimension "d168" = 15
  dimension "d169" = 15
  dimension "d170" = 81
  dimension "d171" = 15
  dimension "d172" = 15
  dimension "d173" = 15
  dimension "d174" = 15
  dimension "d175" = 15
  dimension "d177" = 3
  constraint horizontal L4
  constraint vertical L5
  constraint horizontal L6
  constraint vertical L7
  constraint coincident L2.end L3.start
  constraint horizontal L8
  constraint vertical L9
  constraint horizontal L10
  constraint vertical L11
  constraint horizontal L12
  constraint vertical L13
  constraint horizontal L14
  constraint vertical L15
  constraint horizontal L16
  constraint vertical L17
  constraint horizontal L18
  constraint vertical L19
  constraint horizontal L20
  constraint vertical L21
  constraint horizontal L22
  constraint vertical L23
  constraint horizontal L24
  constraint vertical L25
  constraint horizontal L26
  constraint vertical L27
  constraint horizontal L28
  constraint vertical L29
  constraint horizontal L30
  constraint vertical L31
  constraint horizontal L32
  constraint vertical L33
  constraint horizontal L34
  constraint vertical L35
  constraint horizontal L36
  constraint vertical L37
  constraint horizontal L38
  constraint vertical L39
  constraint horizontal L40
  constraint vertical L41
  constraint horizontal L42
  constraint vertical L43
  constraint horizontal L44
  constraint vertical L45
  constraint horizontal L46
  constraint vertical L47
  constraint horizontal L48
  constraint vertical L49
  constraint horizontal L50
  constraint vertical L51
  constraint horizontal L52
  constraint vertical L53
  constraint horizontal L54
  constraint vertical L55
  constraint horizontal L56
  constraint vertical L57
  constraint horizontal L58
  constraint vertical L59
  constraint horizontal L60
  constraint vertical L61
  constraint horizontal L62
  constraint vertical L63
  constraint horizontal L64
  constraint vertical L65
  constraint horizontal L66
  constraint vertical L67
  constraint horizontal L68
  constraint vertical L69
  constraint horizontal L70
  constraint vertical L71
  constraint horizontal L72
  constraint vertical L73
  constraint horizontal L74
  constraint vertical L75
  constraint horizontal L76
  constraint vertical L77
  constraint horizontal L78
  constraint vertical L79
  constraint horizontal L80
  constraint vertical L81
  constraint horizontal L82
  constraint vertical L83
  constraint horizontal L84
  constraint vertical L85
  constraint horizontal L86
  constraint vertical L87
  constraint horizontal L88
  constraint vertical L89
  constraint horizontal L90
  constraint vertical L91
  constraint horizontal L92
  constraint vertical L93
  constraint horizontal L94
  constraint vertical L95
  constraint horizontal L96
  constraint vertical L97
  constraint horizontal L98
  constraint vertical L99
  constraint horizontal L100
  constraint vertical L101
  constraint horizontal L102
  constraint vertical L103
  constraint coincident L19 L100.start
  constraint coincident L70 L100.start
  constraint horizontal L104
  constraint vertical L105
  constraint horizontal L106
  constraint vertical L107
  constraint coincident L27 L104.start
  constraint coincident L72 L104.start
  constraint horizontal L108
  constraint vertical L109
  constraint horizontal L110
  constraint vertical L111
  constraint coincident L70 L108.start
  constraint coincident L35 L108.start
  constraint horizontal L112
  constraint vertical L113
  constraint horizontal L114
  constraint vertical L115
  constraint coincident L19 L112.start
  constraint coincident L80 L112.start
  constraint horizontal L116
  constraint vertical L117
  constraint horizontal L118
  constraint vertical L119
  constraint coincident L27 L116.start
  constraint coincident L80 L116.start
  constraint horizontal L120
  constraint vertical L121
  constraint horizontal L122
  constraint vertical L123
  constraint coincident L35 L120.start
  constraint coincident L78 L120.start
  constraint horizontal L124
  constraint vertical L125
  constraint horizontal L126
  constraint vertical L127
  constraint coincident L19 L124.start
  constraint coincident L86 L124.start
  constraint horizontal L128
  constraint vertical L129
  constraint horizontal L130
  constraint vertical L131
  constraint coincident L19 L128.start
  constraint coincident L94 L128.start
  constraint horizontal L132
  constraint vertical L133
  constraint horizontal L134
  constraint vertical L135
  constraint coincident L27 L132.start
  constraint coincident L88 L132.start
  constraint horizontal L136
  constraint vertical L137
  constraint horizontal L138
  constraint vertical L139
  constraint coincident L27 L136.start
  constraint coincident L94 L136.start
  constraint horizontal L140
  constraint vertical L141
  constraint horizontal L142
  constraint vertical L143
  constraint coincident L94 L140.start
  constraint coincident L35 L140.start
  constraint horizontal L144
  constraint vertical L145
  constraint horizontal L146
  constraint vertical L147
  constraint coincident L86 L144.start
  constraint coincident L35 L144.start
  constraint horizontal L148
  constraint vertical L149
  constraint horizontal L150
  constraint vertical L151
  constraint horizontal L152
  constraint vertical L153
  constraint horizontal L154
  constraint vertical L155
  constraint horizontal L156
  constraint vertical L157
  constraint horizontal L158
  constraint vertical L159
  constraint horizontal L160
  constraint vertical L161
  constraint horizontal L162
  constraint vertical L163
  constraint coincident L43 L160.start
  constraint coincident L72 L160.start
  constraint horizontal L164
  constraint vertical L165
  constraint horizontal L166
  constraint vertical L167
  constraint coincident L51 L164.start
  constraint coincident L70 L164.start
  constraint horizontal L168
  constraint vertical L169
  constraint horizontal L170
  constraint vertical L171
  constraint coincident L59 L168.start
  constraint coincident L72 L168.start
  constraint horizontal L172
  constraint vertical L173
  constraint horizontal L174
  constraint vertical L175
  constraint coincident L43 L172.start
  constraint coincident L78 L172.start
  constraint horizontal L176
  constraint vertical L177
  constraint horizontal L178
  constraint vertical L179
  constraint coincident L51 L176.start
  constraint coincident L80 L176.start
  constraint horizontal L180
  constraint vertical L181
  constraint horizontal L182
  constraint vertical L183
  constraint coincident L43 L180.start
  constraint coincident L86 L180.start
  constraint horizontal L184
  constraint vertical L185
  constraint horizontal L186
  constraint vertical L187
  constraint coincident L51 L184.start
  constraint coincident L86 L184.start
  constraint horizontal L188
  constraint vertical L189
  constraint horizontal L190
  constraint vertical L191
  constraint coincident L43 L188.start
  constraint coincident L96 L188.start
  constraint horizontal L192
  constraint vertical L193
  constraint horizontal L194
  constraint vertical L195
  constraint coincident L96 L192.start
  constraint coincident L51 L192.start
  constraint horizontal L196
  constraint vertical L197
  constraint horizontal L198
  constraint vertical L199
  constraint coincident L59 L196.start
  constraint coincident L94 L196.start
  constraint horizontal L200
  constraint vertical L201
  constraint horizontal L202
  constraint vertical L203
  constraint coincident L59 L200.start
  constraint coincident L88 L200.start
  constraint horizontal L204
  constraint vertical L205
  constraint horizontal L206
  constraint vertical L207
  constraint horizontal L208
  constraint vertical L209
  constraint horizontal L210
  constraint vertical L211
  constraint horizontal L212
  constraint vertical L213
  constraint horizontal L214
  constraint vertical L215
  constraint coincident L59 L212.start
  constraint coincident L78 L212.start
  constraint horizontal L216
  constraint vertical L217
  constraint horizontal L218
  constraint vertical L219
  constraint horizontal L220
  constraint vertical L221
  constraint horizontal L222
  constraint vertical L223
  constraint horizontal L224
  constraint vertical L225
  constraint horizontal L226
  constraint vertical L227
  constraint horizontal L228
  constraint vertical L229
  constraint horizontal L230
  constraint vertical L231
  constraint horizontal L232
  constraint vertical L233
  constraint horizontal L234
  constraint vertical L235
  constraint horizontal L236
  constraint vertical L237
  constraint horizontal L238
  constraint vertical L239
  constraint coincident L0.end L1.start
  constraint midpoint L148 L240.start
  constraint perpendicular L148 L240
  constraint midpoint L154 P0
  constraint coincident L236 L241.start
  constraint perpendicular L238 L241
  constraint coincident A0.centre L242.start
  constraint perpendicular L68 L242
  constraint midpoint L115 L243.start
  constraint midpoint L113 L243.end
  constraint midpoint L243 P1
  constraint coincident L242 P2
  constraint midpoint L125 L244.start
  constraint midpoint L127 L244.end
  constraint midpoint L129 L245.start
  constraint midpoint L131 L245.end
  constraint midpoint L245 P3
  constraint perpendicular L239 L246
  constraint perpendicular L220 L247
  constraint midpoint L221 A34.centre
  measures "d11" distance of L2.end L4.end
  measures "d12" distance of L4.end L8.end
  measures "d13" distance of L8.end L12.end
  measures "d14" distance of L8.end L14.end
  measures "d15" distance of L12.end L16.end
  measures "d18" distance of L20.end L24.end
  measures "d19" distance of L24.end L28.end
  measures "d20" distance of L24.end L30.end
  measures "d21" distance of L28.end L32.end
  measures "d22" distance of L32.end L36.end
  measures "d23" distance of L32.end L38.end
  measures "d24" distance of L36.end L40.end
  measures "d25" distance of L40.end L44.end
  measures "d26" distance of L40.end L46.end
  measures "d27" distance of L44.end L48.end
  measures "d28" distance of L48.end L52.end
  measures "d29" distance of L48.end L54.end
  measures "d30" distance of L52.end L56.end
  measures "d31" distance of L52.end L58.end
  measures "d32" distance of L56.end L62.end
  measures "d33" distance of L61.end L66.end
  measures "d34" distance of L66.end L70.end
  measures "d35" distance of L70.end L74.end
  measures "d36" distance of L74.end L78.end
  measures "d37" distance of L78.end L82.end
  measures "d38" distance of L82.end L86.end
  measures "d39" distance of L86.end L90.end
  measures "d40" distance of L90.end L94.end
  measures "d41" distance of L94.end L98.end
  measures "d42" distance of L100.start L100.end
  measures "d43" distance of L100.start L102.end